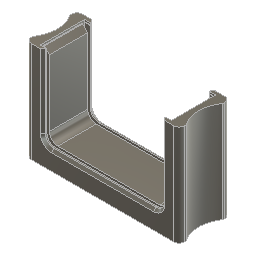
Cuvette 1mm thick (Autodesk Fusion 360 design; units mm, degrees)
Autodesk Fusion 360 part; units mm, degrees
sketch "Sketch1" plane through (0, 0, 0) normal (0, 0, 1) x (1, 0, 0)
  line L0 (0, 0) -> (90, 0)
  line L1 (90, 0) -> (90, 58)
  line L2 (90, 58) -> (0, 58)
  line L3 (0, 58) -> (0, 0)
  line L4 (45, 58) -> (45, 0)
  line L5 (75, 11) -> (15, 11)
  line L6 (10, 16) -> (10, 105)
  line L7 (10, 105) -> (80, 105)
  line L8 (80, 105) -> (80, 16)
  line L9 (80, 11) -> (10, 105) construction
  line L10 (10, 11) -> (80, 105) construction
  arc A0 (10, 16) -> (15, 11) centre (15, 16) ccw
  arc A1 (75, 11) -> (80, 16) centre (75, 16) ccw
  point P0 (45, 58)
  dimension "d1" = 90
  dimension "d2" = 58
  dimension "d3" = 70
  dimension "d5" = 47
  dimension "d6" = 5
  dimension "d7" = 5
  constraint horizontal L0
  constraint vertical L1
  constraint horizontal L2
  constraint vertical L3
  constraint coincident L0.start L3.end
  constraint midpoint L2 P0
  constraint midpoint L0 L4.end
  constraint horizontal L5
  constraint perpendicular L5 L6
  constraint parallel L5 L7
  constraint parallel L6 L8
  constraint coincident L9 P0
  constraint coincident L10 P0
  constraint coincident P0 L4.start
  constraint coincident L10.start L6
  constraint coincident L10.start L5
  constraint tangent L6 A0
  constraint tangent L5 A0
  constraint coincident L9.start L5
  constraint coincident L9.start L8
  constraint tangent L5 A1
  constraint tangent L8 A1
  measures "d1" distance of L0.start L0.end
  measures "d2" distance of L0.start L2.end
  measures "d3" distance of L6.end L7.end
  measures "d5" distance of L2 L5
  measures "d6" radius of A0
  measures "d7" radius of A1
extrude "Extrude1" add sketch "Sketch1" along normal blind 30 contours L0 L2 L3 L4 L5 L6 A0 | L0 L1 L2 L4 L5 L8 A1
sketch "Slide Dimensions" plane through (0, 58, 0) normal (0, 1, 0) x (-1, 0, 0)
  line L0 (-90, 0) -> (-80, 0)
  line L1 (-80, 0) -> (-80, 30)
  line L2 (-80, 30) -> (-90, 30)
  line L3 (-90, 30) -> (-90, 0)
  line L4 (0, 0) -> (-90, 0)
  line L5 (-45, 0) -> (-45, 30.2086)
  line L6 (-83.5, 3.75) -> (-6.5, 3.75)
  line L7 (-6.5, 3.75) -> (-6.5, 2.25)
  line L8 (-6.5, 2.25) -> (-83.5, 2.25)
  line L9 (-83.5, 2.25) -> (-83.5, 3.75)
  line L10 (-83.5, 3.75) -> (-6.5, 2.25) construction
  line L11 (-6.5, 3.75) -> (-83.5, 2.25) construction
  line L12 (0, 30) -> (-90, 30)
  line L13 (-83.5, 27.75) -> (-6.5, 27.75)
  line L14 (-6.5, 27.75) -> (-6.5, 26.25)
  line L15 (-6.5, 26.25) -> (-83.5, 26.25)
  line L16 (-83.5, 26.25) -> (-83.5, 27.75)
  line L17 (-83.5, 27.75) -> (-6.5, 26.25) construction
  line L18 (-6.5, 27.75) -> (-83.5, 26.25) construction
  point P0 (-45, 3)
  point P1 (-45, 27)
  dimension "d10" = 77
  dimension "d11" = 1.5
  dimension "d12" = 3
  dimension "d13" = 77
  dimension "d14" = 1.5
  dimension "d15" = 3
  constraint midpoint L4 L5.start
  constraint perpendicular L4 L5
  constraint horizontal L6
  constraint perpendicular L6 L7
  constraint parallel L6 L8
  constraint parallel L7 L9
  constraint coincident L10 P0
  constraint coincident L11 P0
  constraint coincident L5 P0
  constraint horizontal L13
  constraint perpendicular L13 L14
  constraint parallel L13 L15
  constraint parallel L14 L16
  constraint coincident L17 P1
  constraint coincident L18 P1
  constraint coincident L5 P1
  measures "d10" distance of L7.end L8.end
  measures "d11" distance of L6.end L7.end
  measures "d12" distance of L4 P0
  measures "d13" distance of L14.end L15.end
  measures "d14" distance of L13.end L14.end
  measures "d15" distance of L12 P1
extrude "Extrude2" cut sketch "Slide Dimensions" against normal blind 51 contours L1 L6 L8 L9 | L1 L5 L6 L8 | L5 L6 L7 L8 | L1 L5 L13 L15 | L1 L13 L15 L16 | L5 L13 L14 L15
sketch "Sketch3" plane through (0, 58, 0) normal (0, 1, 0) x (-1, 0, 0)
  line L0 (-10, 3.75) -> (-6.5, 3.75)
  line L1 (-6.5, 3.75) -> (-6.5, 2.25)
  line L2 (-6.5, 2.25) -> (-10, 2.25)
  line L3 (-10, 2.25) -> (-10, 0)
  line L4 (-10, 0) -> (0, 0)
  line L5 (0, 0) -> (0, 30)
  line L6 (0, 30) -> (-10, 30)
  line L7 (-10, 30) -> (-10, 27.75)
  line L8 (-10, 27.75) -> (-6.5, 27.75)
  line L9 (-6.5, 27.75) -> (-6.5, 26.25)
  line L10 (-6.5, 26.25) -> (-10, 26.25)
  line L11 (-10, 26.25) -> (-10, 3.75)
  line L12 (0, 15) -> (-104.5351, 15)
  line L13 (0, 15) -> (23.3341, 15)
  line L14 (-90, 0) -> (-90, 30)
  circle A0 centre (15.6, 15) radius 19
  circle A1 centre (-105.6, 15) radius 19
  dimension "d18" = 38
  dimension "d19" = 15.6
  dimension "d20" = 38
  dimension "d21" = 15.6
  constraint midpoint L5 L12.start
  constraint perpendicular L5 L12
  constraint perpendicular L5 L13
  constraint coincident L13 A0.centre
  constraint coincident L12 A1.centre
  measures "d18" diameter of A0
  measures "d19" distance of L5 A0.centre
  measures "d20" diameter of A1
  measures "d21" distance of L14 A1.centre
extrude "Extrude3" cut sketch "Sketch3" against normal blind 64.145 contours L5 L12 A0 | L5 L12 A0 | L12 L14 A1 | L12 L14 A1
chamfer "Chamfer1" distance 1.5 angle 45 5 edges at (80, 37, 30) (78.5355, 12.4645, 30) (45, 11, 30) (11.4645, 12.4645, 30) (10, 37, 30)
chamfer "Chamfer2" distance 1.5 angle 45 5 edges at (45, 11, 0) (11.4645, 12.4645, 0) (10, 37, 0) (80, 37, 0) (78.5355, 12.4645, 0)
fillet "Fillet1" radius 3 4 edges at (90, 29, 0) (90, 29, 30) (0, 29, 30) (0, 29, 0)
chamfer "Chamfer3" distance 3 angle 45 1 edges at (10, 58, 15)
chamfer "Chamfer3" distance 3 angle 45 1 edges at (80, 58, 15)
sketch "RecessedTopSlide" plane through (0, 58, 0) normal (0, 1, 0) x (-1, 0, 0)
  line L0 (-7, 26.25) -> (-7, 3.75)
  line L1 (-7, 3.75) -> (-6.5, 3.75)
  line L2 (-6.5, 3.75) -> (-6.5, 2.25)
  line L3 (-6.5, 2.25) -> (-10, 2.25)
  line L4 (-10, 2.25) -> (-10, 1.5)
  line L5 (-10, 1.5) -> (-8.5, 0)
  line L6 (-8.5, 0) -> (-3, 0)
  arc A0 (-3, 0) -> (0, 3) centre (-3, 3) ccw
  line L7 (0, 3) -> (0, 4.1538)
  arc A1 (0, 25.8462) -> (0, 4.1538) centre (15.6, 15) ccw
  line L8 (0, 25.8462) -> (0, 27)
  arc A2 (0, 27) -> (-3, 30) centre (-3, 27) ccw
  line L9 (-3, 30) -> (-8.5, 30)
  line L10 (-8.5, 30) -> (-10, 28.5)
  line L11 (-10, 28.5) -> (-10, 27.75)
  line L12 (-10, 27.75) -> (-6.5, 27.75)
  line L13 (-6.5, 27.75) -> (-6.5, 26.25)
  line L14 (-6.5, 26.25) -> (-7, 26.25)
  line L15 (-83.5, 26.25) -> (-6.5, 26.25)
  line L16 (-6.5, 26.25) -> (-6.5, 27.75)
  line L17 (-6.5, 27.75) -> (-83.5, 27.75)
  line L18 (-83.5, 27.75) -> (-83.5, 26.25)
  line L19 (-83.5, 2.25) -> (-6.5, 2.25)
  line L20 (-6.5, 2.25) -> (-6.5, 3.75)
  line L21 (-6.5, 3.75) -> (-83.5, 3.75)
  line L22 (-83.5, 3.75) -> (-83.5, 2.25)
  line L23 (-6.5, 2.25) -> (-83.5, 27.75)
  line L24 (-83.5, 2.25) -> (-6.5, 27.75)
  line L25 (-83.5, 28) -> (-6.5, 28)
  line L26 (-6.5, 28) -> (-6.5, 2)
  line L27 (-6.5, 2) -> (-83.5, 2)
  line L28 (-83.5, 2) -> (-83.5, 28)
  line L29 (-83.5, 28) -> (-6.5, 2) construction
  line L30 (-6.5, 28) -> (-83.5, 2) construction
  line L31 (-83, 3.75) -> (-83, 26.25)
  line L32 (-83, 26.25) -> (-83.5, 26.25)
  line L33 (-83.5, 26.25) -> (-83.5, 27.75)
  line L34 (-83.5, 27.75) -> (-80, 27.75)
  line L35 (-80, 27.75) -> (-80, 28.5)
  line L36 (-80, 28.5) -> (-81.5, 30)
  line L37 (-81.5, 30) -> (-87, 30)
  arc A3 (-87, 30) -> (-90, 27) centre (-87, 27) ccw
  line L38 (-90, 27) -> (-90, 25.8462)
  arc A4 (-90, 4.1538) -> (-90, 25.8462) centre (-105.6, 15) ccw
  line L39 (-90, 4.1538) -> (-90, 3)
  arc A5 (-90, 3) -> (-87, 0) centre (-87, 3) ccw
  line L40 (-87, 0) -> (-81.5, 0)
  line L41 (-81.5, 0) -> (-80, 1.5)
  line L42 (-80, 1.5) -> (-80, 2.25)
  line L43 (-80, 2.25) -> (-83.5, 2.25)
  line L44 (-83.5, 2.25) -> (-83.5, 3.75)
  line L45 (-83.5, 3.75) -> (-83, 3.75)
  point P0 (-45, 15)
  dimension "d30" = 77
  dimension "d31" = 26
  constraint coincident L2.end L3.start
  constraint coincident L17.end L18.start
  constraint coincident L19.start L22.end
  constraint coincident L12.end L13.start
  constraint horizontal L25
  constraint perpendicular L25 L26
  constraint parallel L25 L27
  constraint parallel L26 L28
  constraint coincident L29 P0
  constraint coincident L30 P0
  constraint midpoint L24 P0
  measures "d30" distance of L26.end L27.end
  measures "d31" distance of L25.end L26.end
extrude "Extrude4" add sketch "RecessedTopSlide" along normal blind 1.2 contours L2 L4 L5 L6 A0 L7 A1 L8 A2 L9 L10 L11 L13 L16 L20 L25 L26 L27 | L18 L22 L25 L27 L28 L33 L35 L36 L37 A3 L38 A4 L39 A5 L40 L41 L42 L44
named bodies: "cuvette"
